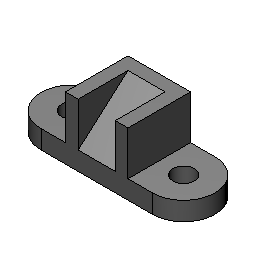
A2 v1 (Autodesk Fusion 360 design; units mm, degrees)
Autodesk Fusion 360 part; units mm, degrees
sketch "Sketch1" plane through (0, 0, 0) normal (0, 0, 1) x (1, 0, 0)
  line L0 (57, 32) -> (-57, 32)
  line L1 (-57, -32) -> (57, -32)
  circle A0 centre (57, 0) radius 11
  circle A1 centre (-57, 0) radius 11
  arc A2 (-57, 32) -> (-57, -32) centre (-57, 0) ccw
  arc A3 (57, -32) -> (57, 32) centre (57, 0) ccw
  dimension "d1" = 114
  dimension "d2" = 64
  dimension "d4" = 32
  dimension "d5" = 22
  dimension "d7" = 32
  dimension "d8" = 22
  constraint horizontal L0
  constraint parallel L0 L1
  constraint concentric A0 A3
  constraint concentric A1 A2
  measures "d1" distance of L1.start L1.end
  measures "d2" distance of L0.end L1.start
  measures "d4" radius of A3
  measures "d5" diameter of A0
  measures "d7" radius of A2
  measures "d8" diameter of A1
extrude "Extrude1" add sketch "Sketch1" along normal blind 19 makes body 1
sketch "Sketch2" plane through (0, 0, 0) normal (0, 1, 0) x (1, 0, 0)
  line L0 (-32, -19) -> (32, -19)
  line L1 (32, -19) -> (32, -64)
  line L2 (32, -64) -> (-32, -64)
  line L3 (-32, -64) -> (-32, -19)
  line L4 (-57, -19) -> (57, -19)
  dimension "d11" = 64
  dimension "d12" = 45
  constraint horizontal L0
  constraint vertical L1
  constraint horizontal L2
  constraint vertical L3
  constraint midpoint L0 L4
  measures "d11" distance of L0.start L0.end
  measures "d12" distance of L0.start L2.end
extrude "Extrude2" add sketch "Sketch2" along normal mid plane 64 separate body makes body 2
sketch "Sketch3" plane through (0, -32, 0) normal (0, -1, 0) x (1, 0, 0)
  line L0 (32, 64) -> (-32, 64)
  line L1 (-32, 64) -> (-32, 19)
  line L2 (-32, 19) -> (32, 19)
  line L3 (32, 19) -> (32, 64)
  line L4 (-19, 64) -> (19, 64)
  line L5 (19, 64) -> (19, 19)
  line L6 (19, 19) -> (-19, 19)
  line L7 (-19, 19) -> (-19, 64)
  dimension "d15" = 38
  dimension "d16" = 45
  constraint horizontal L4
  constraint vertical L5
  constraint horizontal L6
  constraint vertical L7
  constraint coincident L0 L4.start
  constraint midpoint L2 L6
  measures "d15" distance of L4.start L4.end
  measures "d16" distance of L4.start L6.end
extrude "Extrude3" cut sketch "Sketch3" against normal blind 51 contours L0 L2 L4 L5 L6 L7 bodies 2
sketch "Sketch4" plane through (-19, 0, 0) normal (1, 0, 0) x (0, 1, 0)
  line L0 (-32, 64) -> (-32, 19)
  line L1 (-32, 19) -> (19, 19)
  line L2 (19, 19) -> (19, 64)
  line L3 (19, 64) -> (-32, 64)
  line L4 (-32, 19) -> (19, 19)
  line L5 (19, 19) -> (19, 64)
  line L6 (-32, 19) -> (19, 64)
  dimension "d19" = 51
  dimension "d20" = 45
  constraint coincident L0.end L1.start
  constraint coincident L1.end L2.start
  constraint coincident L2.end L3.start
  measures "d19" distance of L0.end L1.end
  measures "d20" distance of L1.end L2.end
extrude "Extrude4" add sketch "Sketch4" along normal blind 38 contours L1 L2 L4 L5 L6 bodies 1 2
equation "d12 = 64 mm - 19 mm"
equation "d16 = 64 mm - 19 mm"
named bodies: "A2"
